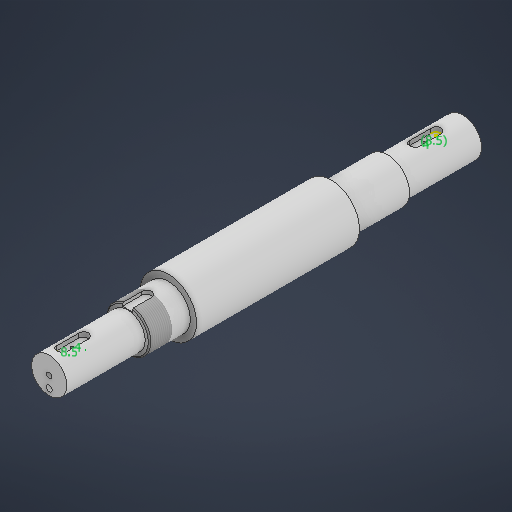
# Autodesk Inventor part: Wał
Saved by Autodesk Inventor 2026 (Build 300175050, 175E)
## iProperties
Created: 2025-06-02
Part Number: Wał
Material: Generic
Document SubType Name: Modeling
Designer: Jan Starachowski
Density: 1 g/cm^3
Appearance: Default
Author: Jan Starachowski
Autodesk Inventor part; units mm, degrees
ref_plane "YZ Plane" through (0, 0, 0) normal (1, 0, 0) x (0, 1, 0)
sketch "Sketch1" plane through (0, 0, 0) normal (1, 0, 0) x (0, 1, 0)
  line L0 (0, 195.7063) -> (0, -134.2937)
  line L1 (0, 195.7063) -> (14, 195.7063)
  line L2 (15, -134.2937) -> (0, -134.2937)
  line L3 (17.5, 100.7063) -> (22.5, 100.7063)
  line L4 (22.5, 100.7063) -> (22.5, -29.2937)
  line L5 (22.5, -29.2937) -> (17.5, -29.2937)
  line L6 (17.5, 100.7063) -> (17.5, 133.2063)
  line L7 (17.5, 133.2063) -> (14, 133.2063)
  line L8 (17.5, -29.2937) -> (17.5, -74.2937)
  line L9 (17.5, -74.2937) -> (15, -74.2937)
  line L10 (14, 195.7063) -> (14, 133.2063)
  line L11 (15, -74.2937) -> (15, -134.2937)
  point P0 (0, 0)
  point P1 (15.75, 133.2063)
  point P2 (20, -29.2937)
  point P3 (7.5, -134.2937)
  point P4 (16.25, -74.2937)
  dimension "d0" = 330
  dimension "d1" = 28
  dimension "d2" = 35
  dimension "d3" = 45
  dimension "d4" = 35
  dimension "d5" = 30
  dimension "d6" = 95
  dimension "d7" = 62.5
  dimension "d8" = 105
  dimension "d9" = 60
  constraints: 24 end point, 13 perpendicular, 4 midpoint, 3 vertical, 1 horizontal
  measures "d0" distance of L0.start L0.end
  measures "d1" diameter of L10 L0
  measures "d2" diameter of L6 L0
  measures "d3" diameter of L4 L0
  measures "d4" diameter of L8 L0
  measures "d5" diameter of L11 L0
  measures "d6" distance from line of L3.end L1
  measures "d7" vertical distance of L1.end point (15.75, 133.206)
  measures "d8" vertical distance of L2.start point (20, -29.294)
  measures "d9" vertical distance of point (7.5, -134.294) point (16.25, -74.294)
revolve "Revolution1" add sketch "Sketch1" angle 360 about axis through (0, 0, 195.7063) along (0, 0, -1)
thread "Thread3" size "M35x1.5" class "6g" standard "ISO Metric profile" length 18
chamfer "Chamfer2" distance 1 angle 45 1 edges at (0, -17.5, 133.2063)
thread "Thread4" size "R 1" standard "ISO Taper" length 23.2
ref_plane "Work Plane1" through (0, 14, 0) normal (0, 1, 0) x (-1, 0, 0)
ref_plane "Work Plane2" through (0, 17.5, 0) normal (0, 1, 0) x (-1, 0, 0)
sketch "Sketch2" plane through (0, 14, 0) normal (0, 1, 0) x (-1, 0, 0)
  line L0 (-14, 195.7063) -> (14, 195.7063) projected
  line L1 (14, 195.7063) -> (14, 133.2063) projected
  line L2 (-14, 195.7063) -> (-14, 133.2063) projected
  line L3 (0, 185.7063) -> (0, 168.7063) construction
  line L4 (-4, 185.7063) -> (-4, 168.7063)
  line L5 (4, 168.7063) -> (4, 185.7063)
  arc A0 (4, 185.7063) -> (-4, 185.7063) centre (0, 185.7063) ccw
  arc A1 (-4, 168.7063) -> (4, 168.7063) centre (0, 168.7063) ccw
  point P0 (0, 0)
  point P1 (0, 177.2063)
  point P2 (0, 164.7063)
  point P3 (0, 189.7063)
  dimension "d29" = 25
  dimension "d30" = 6
  dimension "d31" = 8
  constraints: 8 end point, 6 point on circle, 4 tangent, 2 centre point, 2 parallel, 1 midpoint
  measures "d29" distance of point (0, 164.706) point (0, 189.706)
  measures "d30" distance from line of L0 point (0, 189.706)
  measures "d31" distance between parallel lines of L4 L5
extrude "Extrusion1" cut sketch "Sketch2" against normal blind 4
sketch "Sketch3" plane through (0, 17.5, 0) normal (0, 1, 0) x (-1, 0, 0)
  arc A0 (-4, 118.2063) -> (4, 118.2063) centre (0, 118.2063) ccw
  line L0 (4, 118.2063) -> (4, 133.2938)
  line L1 (-4, 118.2063) -> (-4, 133.2063)
  line L2 (-14, 133.2063) -> (14, 133.2063) projected
  point P0 (0, 0)
  point P1 (0, 114.2063)
  point P2 (0, 133.2063)
  point P3 (4, 133.2063)
  dimension "d34" = 8
  dimension "d35" = 19
  constraints: 4 end point, 3 point on circle, 2 vertical, 1 centre point, 1 midpoint, 1 point on line, 1 tangent
  measures "d34" diameter of A0
  measures "d35" distance of point (0, 114.206) point (0, 133.206)
extrude "Extrusion2" cut sketch "Sketch3" against normal blind 3
ref_plane "Work Plane3" through (0, 15, 0) normal (0, 1, 0) x (-1, 0, 0)
sketch "Sketch4" plane through (0, 15, 0) normal (0, 1, 0) x (-1, 0, 0)
  line L0 (0, -95.7937) -> (0, -112.7937) construction
  line L1 (-4, -95.7937) -> (-4, -112.7937)
  line L2 (4, -112.7937) -> (4, -95.7937)
  arc A0 (4, -95.7937) -> (-4, -95.7937) centre (0, -95.7937) ccw
  arc A1 (-4, -112.7937) -> (4, -112.7937) centre (0, -112.7937) ccw
  line L3 (-15, -134.2937) -> (15, -134.2937) projected
  point P0 (0, 0)
  point P1 (0, -104.2937)
  point P2 (0, -116.7937)
  point P3 (0, -91.7937)
  dimension "d39" = 8
  dimension "d40" = 25
  dimension "d41" = 17.5
  constraints: 8 end point, 6 point on circle, 4 tangent, 2 centre point, 1 midpoint, 1 parallel, 1 vertical
  measures "d39" diameter of A1
  measures "d40" distance of point (0, -116.794) point (0, -91.794)
  measures "d41" distance from line of L3 point (0, -116.794)
extrude "Extrusion3" cut sketch "Sketch4" against normal blind 4
sketch "Sketch11" plane through (0, 11, 0) normal (0, 1, 0) x (1, 0, 0)
  arc A0 (4, 112.7937) -> (-4, 112.7937) centre (0, 112.7937) ccw projected
  line L0 (4, 112.7937) -> (4, 104.2937)
  line L1 (4, 112.7937) -> (4, 95.7937) projected
  line L2 (4, 104.2937) -> (0, 104.2937)
  point P0 (0, 0)
  dimension "d100" = 8.5
  dimension "d101" = 4
  constraints: 4 end point, 1 midpoint, 1 perpendicular
  measures "d100" distance of L0.start L0.end
  measures "d101" distance of L0.end L2.end
sketch "Sketch12" plane through (0, 10, 0) normal (0, 1, 0) x (1, 0, 0)
  arc A0 (-4, -185.7063) -> (4, -185.7063) centre (0, -185.7063) ccw projected
  line L0 (4, -185.7063) -> (4, -177.2063)
  line L1 (4, -177.2063) -> (0, -177.2063)
  point P0 (0, 0)
  dimension "d102" = 8.5
  dimension "d103" = 4
  constraints: 4 end point, 1 perpendicular, 1 tangent, 1 vertical
  measures "d102" distance of L0.start L0.end
  measures "d103" distance of L0.end L1.end
sketch "Sketch5" plane through (0, 0, 195.7063) normal (0, 0, 1) x (1, 0, 0)
  circle A0 centre (0, 0) radius 3
  circle A1 centre (0, -9) radius 2.25
  dimension "d44" = 6
  dimension "d45" = 4.5
  dimension "d46" = 9
  constraints: 2 centre point, 1 coincident
  measures "d44" diameter of A0
  measures "d45" diameter of A1
  measures "d46" distance of A0.centre A1.centre
hole "Hole1" at (0, -9, 195.7063) direction (0, 0, -1) diameter 4.5 depth 12 tip angle 118
sketch "Sketch6" plane through (0, 0, 195.7063) normal (0, 0, 1) x (1, 0, 0)
  circle A0 centre (0, 0) radius 14 projected
  constraints: 1 coincident
hole "Hole2" at (0, 0, 195.7063) direction (0, 0, -1) diameter 4.2 depth 15 tip angle 118
thread "Thread5" size "M5x0.8" class "6H" standard "ISO Metric profile" length 10
sketch "Sketch7" plane through (0, 0, -134.2937) normal (0, 0, -1) x (-1, 0, 0)
  circle A0 centre (0, 0) radius 2.5
  circle A1 centre (0, -9) radius 2.25 projected
  circle A2 centre (0, -9) radius 2.25
  dimension "d63" = 5
  constraints: 2 centre point, 2 coincident
  measures "d63" diameter of A0
hole "Hole3" at (0, -9, -134.2937) direction (0, 0, 1) diameter 4.2 depth 12 tip angle 118
sketch "Sketch8" plane through (0, 0, -134.2937) normal (0, 0, -1) x (-1, 0, 0)
  circle A0 centre (0, 0) radius 15 projected
  constraints: 1 coincident
hole "Hole4" at (0, 0, -134.2937) direction (0, 0, 1) diameter 4 depth 15 tip angle 118
sketch "Sketch9" plane through (0, 10, 0) normal (0, 1, 0) x (1, 0, 0)
  line L0 (4, -168.7063) -> (4, -185.7063) projected
  point P0 (0, 0)
  point P1 (0, -177.2063)
  dimension "d97" = 4
  measures "d97" distance from line of L0 point (0, -177.206)
hole "Hole5" at (0, 10, 177.2063) direction (0, -1, 0) diameter 2.5 depth 7 tip angle 118
thread "Thread7" size "M3x0.5" class "6H" standard "ISO Metric profile" length 6
sketch "Sketch10" plane through (0, 11, 0) normal (0, 1, 0) x (1, 0, 0)
  line L0 (4, 112.7937) -> (4, 95.7937) projected
  point P0 (0, 0)
  point P1 (0, 104.2937)
  dimension "d89" = 4
  measures "d89" distance from line of L0 point (0, 104.294)
hole "Hole6" at (0, 11, -104.2937) direction (0, -1, 0) diameter 2.5 depth 7 tip angle 118
thread "Thread8" size "M3x0.5" class "6H" standard "ISO Metric profile" length 6 offset 1
thread "Thread10" size "M4x0.7" class "6H" standard "ISO Metric profile" length 10
body "Solid1"
